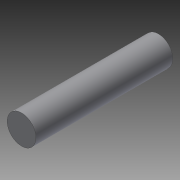
# Autodesk Inventor part: blank
Saved by Autodesk Inventor 2014 SP1 (Build 180222100, 222)
## iProperties
Created: 2015-10-17
Part Number: blank
Material: Generic
Document SubType Name: Modeling
Designer: anthony
Density: 1 g/cm^3
Appearance: Default
Author: anthony
Autodesk Inventor part; units mm, degrees
ref_plane "YZ Plane" through (0, 0, 0) normal (1, 0, 0) x (0, 1, 0)
ref_plane "XZ Plane" through (0, 0, 0) normal (0, 1, 0) x (-1, 0, 0)
ref_plane "XY Plane" through (0, 0, 0) normal (0, 0, 1) x (1, 0, 0)
sketch "Sketch1" plane through (0, 0, 0) normal (0, 1, 0) x (-1, 0, 0)
  circle A0 centre (0, 0) radius 10
  dimension "d0" = 20
  constraints: 1 centre point, 1 coincident
  measures "d0" diameter of A0
extrude "Extrusion1" add sketch "Sketch1" along normal blind 95
shell "Shell1" thickness 1 removed faces 0
sketch "Sketch3" plane through (0, 95, 0) normal (0, 1, 0) x (1, 0, 0)
  circle A0 centre (0, 0) radius 10 projected
  line L0 (-3.1462, 1.4689) -> (3.1462, 1.4689)
  line L1 (4.1462, -0.5311) -> (4.1462, -1.4689)
  line L2 (4.1462, -1.4689) -> (-4.1462, -1.4689)
  line L3 (-4.1462, -1.4689) -> (-4.1462, -0.5311)
  line L4 (-4.1462, 1.4689) -> (4.1462, -1.4689) construction
  line L5 (4.1462, 1.4689) -> (-4.1462, -1.4689) construction
  line L6 (-4.1462, -0.5311) -> (-3.1462, 1.4689)
  line L7 (4.1462, -0.5311) -> (3.1462, 1.4689)
  dimension "d8" = 2
  dimension "d9" = 1
  dimension "d10" = 2
  dimension "d11" = 1
  constraints: 16 end point, 4 point on line, 2 midpoint, 2 parallel, 1 horizontal, 1 perpendicular
  measures "d8" distance of L3.end L4.start
  measures "d9" distance of L0.start L4.start
  measures "d10" distance of L1.start L5.start
  measures "d11" distance of L0.end L5.start
extrude "Extrusion3" cut sketch "Sketch3" against normal blind 5 contours L0 L7 L1 L2 L3 L6
body "Solid1"
